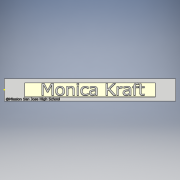
# Autodesk Inventor part: NameTag
Saved by Autodesk Inventor 2018 (Build 220112000, 112)
## iProperties
Created: 2019-03-18
Part Number: NameTag
Material: Generic
Document SubType Name: Modeling
Designer: This kid
Density: 1 g/cm^3
Appearance: Default
Author: This kid
Autodesk Inventor part; units mm, degrees
(part 1 of 2)
ref_plane "YZ Plane" through (0, 0, 0) normal (1, 0, 0) x (0, 1, 0)
ref_plane "XZ Plane" through (0, 0, 0) normal (0, 1, 0) x (-1, 0, 0)
ref_plane "XY Plane" through (0, 0, 0) normal (0, 0, 1) x (1, 0, 0)
sketch "Sketch1" plane through (0, 0, 0) normal (0, 0, 1) x (1, 0, 0)
  line L0 (0, 6.6514) -> (5.7603, -3.3257)
  line L1 (5.7603, -3.3257) -> (-5.7603, -3.3257)
  line L2 (-5.7603, -3.3257) -> (0, 6.6514)
  point P0 (0, 0)
  point P1 (0, 0)
  constraints: 6 end point, 1 coincident, 7 other
extrude "Extrusion1" add sketch "Sketch1" along normal blind 76.2
sketch "Sketch2" plane through (-5.7603, -3.3257, 0) normal (-0.8660254, 0.5, 0) x (0, 0, 1)
  line L0 (9.0292, 2.0917) -> (67.1704, 2.0917)
  line L1 (67.1704, 2.0917) -> (67.1704, 9.2481)
  line L2 (67.1704, 9.2481) -> (9.0292, 9.2481)
  line L3 (9.0292, 9.2481) -> (9.0292, 2.0917)
  line L4 (0, 5.7603) -> (9.0292, 5.6699) construction
  line L5 (67.1704, 5.7603) -> (76.2, 5.7603) construction
  constraints: 12 end point, 2 parallel, 1 equal length, 1 horizontal, 1 midpoint, 1 perpendicular, 1 point on line
extrude "Extrusion2" add sketch "Sketch2" along normal blind 0.2286
sketch "Sketch3" plane through (-5.9582, -3.2114, 0) normal (-0.8660254, 0.5, 0) x (0, 0, 1)
  point P0 (0, 5.7603)
sketch "Sketch4" plane through (-5.9582, -3.2114, 0) normal (-0.8660254, 0.5, 0) x (0, 0, 1)
  line L0 (9.8332, 9.129) -> (68.5929, 9.129) construction
  line L1 (68.5929, 9.129) -> (68.5929, 1.5104) construction
  line L2 (68.5929, 1.5104) -> (9.8332, 1.5104) construction
  line L3 (9.8332, 1.5104) -> (9.8332, 9.129) construction
  line L4 (21.8982, 2.7218) -> (21.0881, 2.7218)
  line L5 (21.0881, 2.7218) -> (21.0881, 7.9731)
  line L6 (21.0881, 7.9731) -> (19.4974, 4.4014)
  line L7 (19.4974, 4.4014) -> (19.0034, 4.4014)
  line L8 (19.0034, 4.4014) -> (17.4275, 7.9731)
  line L9 (17.4275, 7.9731) -> (17.4275, 2.7218)
  line L10 (17.4275, 2.7218) -> (16.6717, 2.7218)
  line L11 (16.6717, 2.7218) -> (16.6717, 8.8178)
  line L12 (16.6717, 8.8178) -> (17.7783, 8.8178)
  line L13 (17.7783, 8.8178) -> (19.2998, 5.424)
  line L14 (19.2998, 5.424) -> (20.7719, 8.8178)
  line L15 (20.7719, 8.8178) -> (21.8982, 8.8178)
  line L16 (21.8982, 8.8178) -> (21.8982, 2.7218)
  spline S0 degree 2 poles (26.8333, 5.009) (26.8333, 3.8531) (25.7218, 2.5934) (24.7931, 2.5934) knots 0 0 0 1 2 2 2
  spline S1 degree 2 poles (24.7931, 2.5934) (23.8397, 2.5934) (22.7479, 3.8926) (22.7479, 5.009) knots 0 0 0 1 2 2 2
  spline S2 degree 2 poles (22.7479, 5.009) (22.7479, 6.1551) (23.8743, 7.4247) (24.7931, 7.4247) knots 0 0 0 1 2 2 2
  spline S3 degree 2 poles (24.7931, 7.4247) (25.7218, 7.4247) (26.8333, 6.1601) (26.8333, 5.009) knots 0 0 0 1 2 2 2
  spline S4 degree 2 poles (26.038, 5.009) (26.038, 5.8983) (25.3908, 6.7628) (24.7931, 6.7628) knots 0 0 0 1 2 2 2
  spline S5 degree 2 poles (24.7931, 6.7628) (24.1954, 6.7628) (23.5433, 5.8983) (23.5433, 5.009) knots 0 0 0 1 2 2 2
  spline S6 degree 2 poles (23.5433, 5.009) (23.5433, 4.1445) (24.1954, 3.2553) (24.7931, 3.2553) knots 0 0 0 1 2 2 2
  spline S7 degree 2 poles (24.7931, 3.2553) (25.3859, 3.2553) (26.038, 4.1297) (26.038, 5.009) knots 0 0 0 1 2 2 2
  line L17 (31.2151, 2.7218) -> (30.4445, 2.7218)
  line L18 (30.4445, 2.7218) -> (30.4445, 5.3301)
  spline S8 degree 2 poles (30.4445, 5.3301) (30.4445, 5.6463) (30.3852, 6.1897) (30.2963, 6.3527) knots 0 0 0 1 2 2 2
  spline S9 degree 2 poles (30.2963, 6.3527) (30.2024, 6.5256) (29.8665, 6.6936) (29.58, 6.6936) knots 0 0 0 1 2 2 2
  spline S10 degree 2 poles (29.58, 6.6936) (29.2935, 6.6936) (28.6858, 6.3873) (28.3944, 6.1403) knots 0 0 0 1 2 2 2
  line L19 (28.3944, 6.1403) -> (28.3944, 2.7218)
  line L20 (28.3944, 2.7218) -> (27.6237, 2.7218)
  line L21 (27.6237, 2.7218) -> (27.6237, 7.2963)
  line L22 (27.6237, 7.2963) -> (28.3944, 7.2963)
  line L23 (28.3944, 7.2963) -> (28.3944, 6.7875)
  spline S11 degree 2 poles (28.3944, 6.7875) (28.7402, 7.0987) (29.4071, 7.4247) (29.7825, 7.4247) knots 0 0 0 1 2 2 2
  spline S12 degree 2 poles (29.7825, 7.4247) (30.4544, 7.4247) (31.2151, 6.5355) (31.2151, 5.6908) knots 0 0 0 1 2 2 2
  line L24 (31.2151, 5.6908) -> (31.2151, 2.7218)
  line L25 (33.0825, 2.7218) -> (32.3118, 2.7218)
  line L26 (32.3118, 2.7218) -> (32.3118, 7.2963)
  line L27 (32.3118, 7.2963) -> (33.0825, 7.2963)
  line L28 (33.0825, 7.2963) -> (33.0825, 2.7218)
  line L29 (33.1368, 8.057) -> (32.2624, 8.057)
  line L30 (32.2624, 8.057) -> (32.2624, 8.8573)
  line L31 (32.2624, 8.8573) -> (33.1368, 8.8573)
  line L32 (33.1368, 8.8573) -> (33.1368, 8.057)
  spline S13 degree 2 poles (36.0317, 2.6181) (35.5574, 2.6181) (34.772, 2.9095) (34.4904, 3.2059) knots 0 0 0 1 2 2 2
  spline S14 degree 2 poles (34.4904, 3.2059) (34.2088, 3.4974) (33.8976, 4.3965) (33.8976, 4.9992) knots 0 0 0 1 2 2 2
  spline S15 degree 2 poles (33.8976, 4.9992) (33.8976, 5.6019) (34.2187, 6.4812) (34.4904, 6.7776) knots 0 0 0 1 2 2 2
  spline S16 degree 2 poles (34.4904, 6.7776) (34.7621, 7.0789) (35.5673, 7.4) (36.0317, 7.4) knots 0 0 0 1 2 2 2
  spline S17 degree 2 poles (36.0317, 7.4) (36.4071, 7.4) (37.1086, 7.1876) (37.3803, 7.0493) knots 0 0 0 1 2 2 2
  line L33 (37.3803, 7.0493) -> (37.3803, 6.1848)
  line L34 (37.3803, 6.1848) -> (37.3358, 6.1848)
  spline S18 degree 2 poles (37.3358, 6.1848) (37.2519, 6.2539) (36.995, 6.4318) (36.8122, 6.5256) knots 0 0 0 1 2 2 2
  spline S19 degree 2 poles (36.8122, 6.5256) (36.6492, 6.6047) (36.2145, 6.7282) (36.0169, 6.7282) knots 0 0 0 1 2 2 2
  spline S20 degree 2 poles (36.0169, 6.7282) (35.4191, 6.7282) (34.6929, 5.8242) (34.6929, 4.9992) knots 0 0 0 1 2 2 2
  spline S21 degree 2 poles (34.6929, 4.9992) (34.6929, 4.1939) (35.3944, 3.2899) (36.0169, 3.2899) knots 0 0 0 1 2 2 2
  spline S22 degree 2 poles (36.0169, 3.2899) (36.3923, 3.2899) (37.074, 3.6011) (37.3358, 3.8432) knots 0 0 0 1 2 2 2
  line L35 (37.3358, 3.8432) -> (37.3803, 3.8432)
  line L36 (37.3803, 3.8432) -> (37.3803, 2.9787)
  spline S23 degree 2 poles (37.3803, 2.9787) (37.2667, 2.9244) (36.9209, 2.7712) (36.7826, 2.7366) knots 0 0 0 1 2 2 2
  spline S24 degree 2 poles (36.7826, 2.7366) (36.585, 2.6774) (36.2737, 2.6181) (36.0317, 2.6181) knots 0 0 0 1 2 2 2
  spline S25 degree 2 poles (40.6308, 3.2059) (40.537, 3.1368) (40.2208, 2.8898) (40.0726, 2.8157) knots 0 0 0 1 2 2 2
  spline S26 degree 2 poles (40.0726, 2.8157) (39.8701, 2.707) (39.4897, 2.5934) (39.1439, 2.5934) knots 0 0 0 1 2 2 2
  spline S27 degree 2 poles (39.1439, 2.5934) (38.8623, 2.5934) (38.3535, 2.8058) (38.1608, 2.9985) knots 0 0 0 1 2 2 2
  spline S28 degree 2 poles (38.1608, 2.9985) (37.978, 3.1862) (37.7557, 3.7395) (37.7557, 4.0457) knots 0 0 0 1 2 2 2
  spline S29 degree 2 poles (37.7557, 4.0457) (37.7557, 4.52) (38.1559, 5.1918) (38.5906, 5.3845) knots 0 0 0 1 2 2 2
  spline S30 degree 2 poles (38.5906, 5.3845) (38.9759, 5.5623) (40.0232, 5.6957) (40.6308, 5.7303) knots 0 0 0 1 2 2 2
  line L37 (40.6308, 5.7303) -> (40.6308, 5.8785)
  spline S31 degree 2 poles (40.6308, 5.8785) (40.6308, 6.1453) (40.4678, 6.4762) (40.3196, 6.5701) knots 0 0 0 1 2 2 2
  spline S32 degree 2 poles (40.3196, 6.5701) (40.1714, 6.664) (39.7466, 6.7232) (39.5193, 6.7232) knots 0 0 0 1 2 2 2
  spline S33 degree 2 poles (39.5193, 6.7232) (39.2526, 6.7232) (38.5313, 6.5652) (38.1707, 6.412) knots 0 0 0 1 2 2 2
  line L38 (38.1707, 6.412) -> (38.1263, 6.412)
  line L39 (38.1263, 6.412) -> (38.1263, 7.1975)
  spline S34 degree 2 poles (38.1263, 7.1975) (38.3387, 7.2568) (39.134, 7.405) (39.5243, 7.405) knots 0 0 0 1 2 2 2
  spline S35 degree 2 poles (39.5243, 7.405) (39.9985, 7.405) (40.6457, 7.2568) (40.9025, 7.0641) knots 0 0 0 1 2 2 2
  spline S36 degree 2 poles (40.9025, 7.0641) (41.1545, 6.8764) (41.4015, 6.2786) (41.4015, 5.8489) knots 0 0 0 1 2 2 2
  line L40 (41.4015, 5.8489) -> (41.4015, 2.7218)
  line L41 (41.4015, 2.7218) -> (40.6308, 2.7218)
  line L42 (40.6308, 2.7218) -> (40.6308, 3.2059)
  line L43 (40.6308, 3.8481) -> (40.6308, 5.1177)
  spline S37 degree 2 poles (40.6308, 5.1177) (40.3542, 5.093) (39.5193, 5.009) (39.2575, 4.93) knots 0 0 0 1 2 2 2
  spline S38 degree 2 poles (39.2575, 4.93) (38.9512, 4.8361) (38.5511, 4.4459) (38.5511, 4.1001) knots 0 0 0 1 2 2 2
  spline S39 degree 2 poles (38.5511, 4.1001) (38.5511, 3.7049) (38.9957, 3.3047) (39.4205, 3.3047) knots 0 0 0 1 2 2 2
  spline S40 degree 2 poles (39.4205, 3.3047) (39.7812, 3.3047) (40.374, 3.616) (40.6308, 3.8481) knots 0 0 0 1 2 2 2
  line L44 (49.6069, 2.7218) -> (48.5547, 2.7218)
  line L45 (48.5547, 2.7218) -> (46.3267, 5.5574)
  line L46 (46.3267, 5.5574) -> (45.971, 5.1572)
  line L47 (45.971, 5.1572) -> (45.971, 2.7218)
  line L48 (45.971, 2.7218) -> (45.1609, 2.7218)
  line L49 (45.1609, 2.7218) -> (45.1609, 8.8178)
  line L50 (45.1609, 8.8178) -> (45.971, 8.8178)
  line L51 (45.971, 8.8178) -> (45.971, 6.0168)
  line L52 (45.971, 6.0168) -> (48.4707, 8.8178)
  line L53 (48.4707, 8.8178) -> (49.4587, 8.8178)
  line L54 (49.4587, 8.8178) -> (46.9343, 6.0959)
  line L55 (46.9343, 6.0959) -> (49.6069, 2.7218)
  line L56 (52.4573, 6.4713) -> (52.4178, 6.4713)
  spline S41 degree 2 poles (52.4178, 6.4713) (52.3288, 6.496) (52.1362, 6.5059) (52.0028, 6.5059) knots 0 0 0 1 2 2 2
  spline S42 degree 2 poles (52.0028, 6.5059) (51.6916, 6.5059) (51.079, 6.2342) (50.8024, 5.9674) knots 0 0 0 1 2 2 2
  line L57 (50.8024, 5.9674) -> (50.8024, 2.7218)
  line L58 (50.8024, 2.7218) -> (50.0317, 2.7218)
  line L59 (50.0317, 2.7218) -> (50.0317, 7.2963)
  line L60 (50.0317, 7.2963) -> (50.8024, 7.2963)
  line L61 (50.8024, 7.2963) -> (50.8024, 6.6146)
  spline S43 degree 2 poles (50.8024, 6.6146) (51.2223, 6.99) (51.8497, 7.2963) (52.1461, 7.2963) knots 0 0 0 1 2 2 2
  spline S44 degree 2 poles (52.1461, 7.2963) (52.2646, 7.2963) (52.3832, 7.2864) (52.4573, 7.2716) knots 0 0 0 1 2 2 2
  line L62 (52.4573, 7.2716) -> (52.4573, 6.4713)
  spline S45 degree 2 poles (55.6041, 3.2059) (55.5102, 3.1368) (55.1941, 2.8898) (55.0459, 2.8157) knots 0 0 0 1 2 2 2
  spline S46 degree 2 poles (55.0459, 2.8157) (54.8433, 2.707) (54.4629, 2.5934) (54.1171, 2.5934) knots 0 0 0 1 2 2 2
  spline S47 degree 2 poles (54.1171, 2.5934) (53.8356, 2.5934) (53.3267, 2.8058) (53.1341, 2.9985) knots 0 0 0 1 2 2 2
  spline S48 degree 2 poles (53.1341, 2.9985) (52.9513, 3.1862) (52.729, 3.7395) (52.729, 4.0457) knots 0 0 0 1 2 2 2
  spline S49 degree 2 poles (52.729, 4.0457) (52.729, 4.52) (53.1291, 5.1918) (53.5639, 5.3845) knots 0 0 0 1 2 2 2
  spline S50 degree 2 poles (53.5639, 5.3845) (53.9492, 5.5623) (54.9965, 5.6957) (55.6041, 5.7303) knots 0 0 0 1 2 2 2
  line L63 (55.6041, 5.7303) -> (55.6041, 5.8785)
  spline S51 degree 2 poles (55.6041, 5.8785) (55.6041, 6.1453) (55.4411, 6.4762) (55.2929, 6.5701) knots 0 0 0 1 2 2 2
  spline S52 degree 2 poles (55.2929, 6.5701) (55.1447, 6.664) (54.7198, 6.7232) (54.4926, 6.7232) knots 0 0 0 1 2 2 2
  spline S53 degree 2 poles (54.4926, 6.7232) (54.2258, 6.7232) (53.5046, 6.5652) (53.1439, 6.412) knots 0 0 0 1 2 2 2
  line L64 (53.1439, 6.412) -> (53.0995, 6.412)
  line L65 (53.0995, 6.412) -> (53.0995, 7.1975)
  spline S54 degree 2 poles (53.0995, 7.1975) (53.3119, 7.2568) (54.1073, 7.405) (54.4975, 7.405) knots 0 0 0 1 2 2 2
  spline S55 degree 2 poles (54.4975, 7.405) (54.9718, 7.405) (55.6189, 7.2568) (55.8758, 7.0641) knots 0 0 0 1 2 2 2
  spline S56 degree 2 poles (55.8758, 7.0641) (56.1277, 6.8764) (56.3747, 6.2786) (56.3747, 5.8489) knots 0 0 0 1 2 2 2
  line L66 (56.3747, 5.8489) -> (56.3747, 2.7218)
  line L67 (56.3747, 2.7218) -> (55.6041, 2.7218)
  line L68 (55.6041, 2.7218) -> (55.6041, 3.2059)
  line L69 (55.6041, 3.8481) -> (55.6041, 5.1177)
  spline S57 degree 2 poles (55.6041, 5.1177) (55.3274, 5.093) (54.4926, 5.009) (54.2308, 4.93) knots 0 0 0 1 2 2 2
  spline S58 degree 2 poles (54.2308, 4.93) (53.9245, 4.8361) (53.5243, 4.4459) (53.5243, 4.1001) knots 0 0 0 1 2 2 2
  spline S59 degree 2 poles (53.5243, 4.1001) (53.5243, 3.7049) (53.9689, 3.3047) (54.3938, 3.3047) knots 0 0 0 1 2 2 2
  spline S60 degree 2 poles (54.3938, 3.3047) (54.7544, 3.3047) (55.3472, 3.616) (55.6041, 3.8481) knots 0 0 0 1 2 2 2
  line L70 (59.8624, 8.3485) -> (59.8229, 8.3485)
  spline S61 degree 2 poles (59.8229, 8.3485) (59.7191, 8.388) (59.3338, 8.4572) (59.1807, 8.4572) knots 0 0 0 1 2 2 2
  spline S62 degree 2 poles (59.1807, 8.4572) (58.6965, 8.4572) (58.2816, 8.0225) (58.2816, 7.4494) knots 0 0 0 1 2 2 2
  line L71 (58.2816, 7.4494) -> (58.2816, 7.2963)
  line L72 (58.2816, 7.2963) -> (59.5561, 7.2963)
  line L73 (59.5561, 7.2963) -> (59.5561, 6.659)
  line L74 (59.5561, 6.659) -> (58.3063, 6.659)
  line L75 (58.3063, 6.659) -> (58.3063, 2.7218)
  line L76 (58.3063, 2.7218) -> (57.5356, 2.7218)
  line L77 (57.5356, 2.7218) -> (57.5356, 6.659)
  line L78 (57.5356, 6.659) -> (57.0169, 6.659)
  line L79 (57.0169, 6.659) -> (57.0169, 7.2963)
  line L80 (57.0169, 7.2963) -> (57.5356, 7.2963)
  line L81 (57.5356, 7.2963) -> (57.5356, 7.4494)
  spline S63 degree 2 poles (57.5356, 7.4494) (57.5356, 8.2695) (58.331, 9.129) (59.072, 9.129) knots 0 0 0 1 2 2 2
  spline S64 degree 2 poles (59.072, 9.129) (59.2844, 9.129) (59.6944, 9.0846) (59.8624, 9.0549) knots 0 0 0 1 2 2 2
  line L82 (59.8624, 9.0549) -> (59.8624, 8.3485)
  spline S65 degree 2 poles (61.5074, 2.6329) (60.88, 2.6329) (60.1736, 3.3492) (60.1736, 4.1248) knots 0 0 0 1 2 2 2
  line L83 (60.1736, 4.1248) -> (60.1736, 6.659)
  line L84 (60.1736, 6.659) -> (59.6549, 6.659)
  line L85 (59.6549, 6.659) -> (59.6549, 7.2963)
  line L86 (59.6549, 7.2963) -> (60.1736, 7.2963)
  line L87 (60.1736, 7.2963) -> (60.1736, 8.6103)
  line L88 (60.1736, 8.6103) -> (60.9443, 8.6103)
  line L89 (60.9443, 8.6103) -> (60.9443, 7.2963)
  line L90 (60.9443, 7.2963) -> (62.362, 7.2963)
  line L91 (62.362, 7.2963) -> (62.362, 6.659)
  line L92 (62.362, 6.659) -> (60.9443, 6.659)
  line L93 (60.9443, 6.659) -> (60.9443, 4.4805)
  spline S66 degree 2 poles (60.9443, 4.4805) (60.9443, 4.1347) (60.969, 3.7543) (61.0529, 3.5913) knots 0 0 0 1 2 2 2
  spline S67 degree 2 poles (61.0529, 3.5913) (61.1221, 3.448) (61.4333, 3.3047) (61.7001, 3.3047) knots 0 0 0 1 2 2 2
  spline S68 degree 2 poles (61.7001, 3.3047) (61.8878, 3.3047) (62.2385, 3.4184) (62.3176, 3.4529) knots 0 0 0 1 2 2 2
  line L94 (62.3176, 3.4529) -> (62.362, 3.4529)
  line L95 (62.362, 3.4529) -> (62.362, 2.7613)
  spline S69 degree 2 poles (62.362, 2.7613) (62.1447, 2.7021) (61.7001, 2.6329) (61.5074, 2.6329) knots 0 0 0 1 2 2 2
  point P0 (0, 5.7603)
  constraints: 2 other
extrude "Extrusion3" add sketch "Sketch4" along normal blind 0.254
sketch "Sketch5" plane through (0, 6.6514, 76.2) normal (0.8660254, 0.5, 0) x (0, 0, -1)
  line L0 (67.0697, -2.2328) -> (67.0697, -9.3892)
  line L1 (9.3366, -9.3892) -> (67.0697, -9.3892)
  line L2 (67.0697, -2.2328) -> (9.3366, -2.2328)
  line L3 (9.3366, -2.2328) -> (9.3366, -9.3892)
  line L4 (67.0697, -5.811) -> (76.4063, -5.811) construction
  line L5 (0, -5.7603) -> (9.3366, -5.7603) construction
  constraints: 12 end point, 1 horizontal, 1 midpoint, 1 parallel, 1 perpendicular, 1 point on line, 1 vertical
extrude "Extrusion4" add sketch "Sketch5" along normal blind 0.2286
sketch "Sketch6" plane through (0.198, 6.7657, 76.2) normal (0.8660254, 0.5, 0) x (0, 0, -1)
  line L0 (9.5837, -2.534) -> (68.3434, -2.534) construction
  line L1 (68.3434, -2.534) -> (68.3434, -8.4681) construction
  line L2 (68.3434, -8.4681) -> (9.5837, -8.4681) construction
  line L3 (9.5837, -8.4681) -> (9.5837, -2.534) construction
  line L4 (21.6488, -8.9412) -> (20.8386, -8.9412)
  line L5 (20.8386, -8.9412) -> (20.8386, -3.69)
  line L6 (20.8386, -3.69) -> (19.2479, -7.2616)
  line L7 (19.2479, -7.2616) -> (18.7539, -7.2616)
  line L8 (18.7539, -7.2616) -> (17.1781, -3.69)
  line L9 (17.1781, -3.69) -> (17.1781, -8.9412)
  line L10 (17.1781, -8.9412) -> (16.4222, -8.9412)
  line L11 (16.4222, -8.9412) -> (16.4222, -2.8452)
  line L12 (16.4222, -2.8452) -> (17.5288, -2.8452)
  line L13 (17.5288, -2.8452) -> (19.0503, -6.239)
  line L14 (19.0503, -6.239) -> (20.5225, -2.8452)
  line L15 (20.5225, -2.8452) -> (21.6488, -2.8452)
  line L16 (21.6488, -2.8452) -> (21.6488, -8.9412)
  spline S0 degree 2 poles (26.5839, -6.654) (26.5839, -7.81) (25.4724, -9.0697) (24.5436, -9.0697) knots 0 0 0 1 2 2 2
  spline S1 degree 2 poles (24.5436, -9.0697) (23.5902, -9.0697) (22.4985, -7.7704) (22.4985, -6.654) knots 0 0 0 1 2 2 2
  spline S2 degree 2 poles (22.4985, -6.654) (22.4985, -5.5079) (23.6248, -4.2383) (24.5436, -4.2383) knots 0 0 0 1 2 2 2
  spline S3 degree 2 poles (24.5436, -4.2383) (25.4724, -4.2383) (26.5839, -5.503) (26.5839, -6.654) knots 0 0 0 1 2 2 2
  spline S4 degree 2 poles (25.7885, -6.654) (25.7885, -5.7648) (25.1414, -4.9003) (24.5436, -4.9003) knots 0 0 0 1 2 2 2
  spline S5 degree 2 poles (24.5436, -4.9003) (23.9459, -4.9003) (23.2938, -5.7648) (23.2938, -6.654) knots 0 0 0 1 2 2 2
  spline S6 degree 2 poles (23.2938, -6.654) (23.2938, -7.5185) (23.9459, -8.4077) (24.5436, -8.4077) knots 0 0 0 1 2 2 2
  spline S7 degree 2 poles (24.5436, -8.4077) (25.1364, -8.4077) (25.7885, -7.5333) (25.7885, -6.654) knots 0 0 0 1 2 2 2
  line L17 (30.9657, -8.9412) -> (30.195, -8.9412)
  line L18 (30.195, -8.9412) -> (30.195, -6.3329)
  spline S8 degree 2 poles (30.195, -6.3329) (30.195, -6.0167) (30.1358, -5.4733) (30.0468, -5.3103) knots 0 0 0 1 2 2 2
  spline S9 degree 2 poles (30.0468, -5.3103) (29.953, -5.1374) (29.6171, -4.9694) (29.3305, -4.9694) knots 0 0 0 1 2 2 2
  spline S10 degree 2 poles (29.3305, -4.9694) (29.044, -4.9694) (28.4364, -5.2757) (28.1449, -5.5227) knots 0 0 0 1 2 2 2
  line L19 (28.1449, -5.5227) -> (28.1449, -8.9412)
  line L20 (28.1449, -8.9412) -> (27.3743, -8.9412)
  line L21 (27.3743, -8.9412) -> (27.3743, -4.3668)
  line L22 (27.3743, -4.3668) -> (28.1449, -4.3668)
  line L23 (28.1449, -4.3668) -> (28.1449, -4.8756)
  spline S11 degree 2 poles (28.1449, -4.8756) (28.4907, -4.5644) (29.1576, -4.2383) (29.5331, -4.2383) knots 0 0 0 1 2 2 2
  spline S12 degree 2 poles (29.5331, -4.2383) (30.2049, -4.2383) (30.9657, -5.1275) (30.9657, -5.9723) knots 0 0 0 1 2 2 2
  line L24 (30.9657, -5.9723) -> (30.9657, -8.9412)
  line L25 (32.833, -8.9412) -> (32.0624, -8.9412)
  line L26 (32.0624, -8.9412) -> (32.0624, -4.3668)
  line L27 (32.0624, -4.3668) -> (32.833, -4.3668)
  line L28 (32.833, -4.3668) -> (32.833, -8.9412)
  line L29 (32.8874, -3.606) -> (32.013, -3.606)
  line L30 (32.013, -3.606) -> (32.013, -2.8057)
  line L31 (32.013, -2.8057) -> (32.8874, -2.8057)
  line L32 (32.8874, -2.8057) -> (32.8874, -3.606)
  spline S13 degree 2 poles (35.7822, -9.045) (35.308, -9.045) (34.5225, -8.7535) (34.2409, -8.4571) knots 0 0 0 1 2 2 2
  spline S14 degree 2 poles (34.2409, -8.4571) (33.9593, -8.1656) (33.6481, -7.2666) (33.6481, -6.6639) knots 0 0 0 1 2 2 2
  spline S15 degree 2 poles (33.6481, -6.6639) (33.6481, -6.0612) (33.9692, -5.1819) (34.2409, -4.8855) knots 0 0 0 1 2 2 2
  spline S16 degree 2 poles (34.2409, -4.8855) (34.5126, -4.5841) (35.3179, -4.263) (35.7822, -4.263) knots 0 0 0 1 2 2 2
  spline S17 degree 2 poles (35.7822, -4.263) (36.1577, -4.263) (36.8591, -4.4754) (37.1308, -4.6138) knots 0 0 0 1 2 2 2
  line L33 (37.1308, -4.6138) -> (37.1308, -5.4783)
  line L34 (37.1308, -5.4783) -> (37.0864, -5.4783)
  spline S18 degree 2 poles (37.0864, -5.4783) (37.0024, -5.4091) (36.7455, -5.2313) (36.5627, -5.1374) knots 0 0 0 1 2 2 2
  spline S19 degree 2 poles (36.5627, -5.1374) (36.3997, -5.0584) (35.965, -4.9349) (35.7674, -4.9349) knots 0 0 0 1 2 2 2
  spline S20 degree 2 poles (35.7674, -4.9349) (35.1697, -4.9349) (34.4435, -5.8389) (34.4435, -6.6639) knots 0 0 0 1 2 2 2
  spline S21 degree 2 poles (34.4435, -6.6639) (34.4435, -7.4691) (35.145, -8.3731) (35.7674, -8.3731) knots 0 0 0 1 2 2 2
  spline S22 degree 2 poles (35.7674, -8.3731) (36.1428, -8.3731) (36.8246, -8.0619) (37.0864, -7.8198) knots 0 0 0 1 2 2 2
  line L35 (37.0864, -7.8198) -> (37.1308, -7.8198)
  line L36 (37.1308, -7.8198) -> (37.1308, -8.6843)
  spline S23 degree 2 poles (37.1308, -8.6843) (37.0172, -8.7387) (36.6714, -8.8918) (36.5331, -8.9264) knots 0 0 0 1 2 2 2
  spline S24 degree 2 poles (36.5331, -8.9264) (36.3355, -8.9857) (36.0243, -9.045) (35.7822, -9.045) knots 0 0 0 1 2 2 2
  spline S25 degree 2 poles (40.3814, -8.4571) (40.2875, -8.5263) (39.9714, -8.7733) (39.8232, -8.8474) knots 0 0 0 1 2 2 2
  spline S26 degree 2 poles (39.8232, -8.8474) (39.6206, -8.9561) (39.2402, -9.0697) (38.8944, -9.0697) knots 0 0 0 1 2 2 2
  spline S27 degree 2 poles (38.8944, -9.0697) (38.6129, -9.0697) (38.104, -8.8573) (37.9114, -8.6646) knots 0 0 0 1 2 2 2
  spline S28 degree 2 poles (37.9114, -8.6646) (37.7286, -8.4769) (37.5063, -7.9236) (37.5063, -7.6173) knots 0 0 0 1 2 2 2
  spline S29 degree 2 poles (37.5063, -7.6173) (37.5063, -7.1431) (37.9064, -6.4712) (38.3412, -6.2786) knots 0 0 0 1 2 2 2
  spline S30 degree 2 poles (38.3412, -6.2786) (38.7265, -6.1007) (39.7738, -5.9673) (40.3814, -5.9328) knots 0 0 0 1 2 2 2
  line L37 (40.3814, -5.9328) -> (40.3814, -5.7846)
  spline S31 degree 2 poles (40.3814, -5.7846) (40.3814, -5.5178) (40.2184, -5.1868) (40.0702, -5.0929) knots 0 0 0 1 2 2 2
  spline S32 degree 2 poles (40.0702, -5.0929) (39.922, -4.9991) (39.4971, -4.9398) (39.2699, -4.9398) knots 0 0 0 1 2 2 2
  spline S33 degree 2 poles (39.2699, -4.9398) (39.0031, -4.9398) (38.2819, -5.0979) (37.9212, -5.251) knots 0 0 0 1 2 2 2
  line L38 (37.9212, -5.251) -> (37.8768, -5.251)
  line L39 (37.8768, -5.251) -> (37.8768, -4.4656)
  spline S34 degree 2 poles (37.8768, -4.4656) (38.0892, -4.4063) (38.8846, -4.2581) (39.2748, -4.2581) knots 0 0 0 1 2 2 2
  spline S35 degree 2 poles (39.2748, -4.2581) (39.7491, -4.2581) (40.3962, -4.4063) (40.6531, -4.5989) knots 0 0 0 1 2 2 2
  spline S36 degree 2 poles (40.6531, -4.5989) (40.905, -4.7867) (41.152, -5.3844) (41.152, -5.8142) knots 0 0 0 1 2 2 2
  line L40 (41.152, -5.8142) -> (41.152, -8.9412)
  line L41 (41.152, -8.9412) -> (40.3814, -8.9412)
  line L42 (40.3814, -8.9412) -> (40.3814, -8.4571)
  line L43 (40.3814, -7.8149) -> (40.3814, -6.5453)
  spline S37 degree 2 poles (40.3814, -6.5453) (40.1047, -6.57) (39.2699, -6.654) (39.0081, -6.733) knots 0 0 0 1 2 2 2
  spline S38 degree 2 poles (39.0081, -6.733) (38.7018, -6.8269) (38.3016, -7.2172) (38.3016, -7.563) knots 0 0 0 1 2 2 2
  spline S39 degree 2 poles (38.3016, -7.563) (38.3016, -7.9582) (38.7462, -8.3583) (39.1711, -8.3583) knots 0 0 0 1 2 2 2
  spline S40 degree 2 poles (39.1711, -8.3583) (39.5317, -8.3583) (40.1245, -8.0471) (40.3814, -7.8149) knots 0 0 0 1 2 2 2
  line L44 (49.3574, -8.9412) -> (48.3052, -8.9412)
  line L45 (48.3052, -8.9412) -> (46.0772, -6.1057)
  line L46 (46.0772, -6.1057) -> (45.7216, -6.5058)
  line L47 (45.7216, -6.5058) -> (45.7216, -8.9412)
  line L48 (45.7216, -8.9412) -> (44.9114, -8.9412)
  line L49 (44.9114, -8.9412) -> (44.9114, -2.8452)
  line L50 (44.9114, -2.8452) -> (45.7216, -2.8452)
  line L51 (45.7216, -2.8452) -> (45.7216, -5.6462)
  line L52 (45.7216, -5.6462) -> (48.2212, -2.8452)
  line L53 (48.2212, -2.8452) -> (49.2092, -2.8452)
  line L54 (49.2092, -2.8452) -> (46.6849, -5.5672)
  line L55 (46.6849, -5.5672) -> (49.3574, -8.9412)
  line L56 (52.2078, -5.1917) -> (52.1683, -5.1917)
  spline S41 degree 2 poles (52.1683, -5.1917) (52.0794, -5.167) (51.8867, -5.1572) (51.7533, -5.1572) knots 0 0 0 1 2 2 2
  spline S42 degree 2 poles (51.7533, -5.1572) (51.4421, -5.1572) (50.8296, -5.4289) (50.5529, -5.6956) knots 0 0 0 1 2 2 2
  line L57 (50.5529, -5.6956) -> (50.5529, -8.9412)
  line L58 (50.5529, -8.9412) -> (49.7823, -8.9412)
  line L59 (49.7823, -8.9412) -> (49.7823, -4.3668)
  line L60 (49.7823, -4.3668) -> (50.5529, -4.3668)
  line L61 (50.5529, -4.3668) -> (50.5529, -5.0485)
  spline S43 degree 2 poles (50.5529, -5.0485) (50.9728, -4.673) (51.6002, -4.3668) (51.8966, -4.3668) knots 0 0 0 1 2 2 2
  spline S44 degree 2 poles (51.8966, -4.3668) (52.0152, -4.3668) (52.1337, -4.3766) (52.2078, -4.3915) knots 0 0 0 1 2 2 2
  line L62 (52.2078, -4.3915) -> (52.2078, -5.1917)
  spline S45 degree 2 poles (55.3546, -8.4571) (55.2608, -8.5263) (54.9446, -8.7733) (54.7964, -8.8474) knots 0 0 0 1 2 2 2
  spline S46 degree 2 poles (54.7964, -8.8474) (54.5939, -8.9561) (54.2135, -9.0697) (53.8677, -9.0697) knots 0 0 0 1 2 2 2
  spline S47 degree 2 poles (53.8677, -9.0697) (53.5861, -9.0697) (53.0773, -8.8573) (52.8846, -8.6646) knots 0 0 0 1 2 2 2
  spline S48 degree 2 poles (52.8846, -8.6646) (52.7018, -8.4769) (52.4795, -7.9236) (52.4795, -7.6173) knots 0 0 0 1 2 2 2
  spline S49 degree 2 poles (52.4795, -7.6173) (52.4795, -7.1431) (52.8797, -6.4712) (53.3144, -6.2786) knots 0 0 0 1 2 2 2
  spline S50 degree 2 poles (53.3144, -6.2786) (53.6997, -6.1007) (54.747, -5.9673) (55.3546, -5.9328) knots 0 0 0 1 2 2 2
  line L63 (55.3546, -5.9328) -> (55.3546, -5.7846)
  spline S51 degree 2 poles (55.3546, -5.7846) (55.3546, -5.5178) (55.1916, -5.1868) (55.0434, -5.0929) knots 0 0 0 1 2 2 2
  spline S52 degree 2 poles (55.0434, -5.0929) (54.8952, -4.9991) (54.4704, -4.9398) (54.2431, -4.9398) knots 0 0 0 1 2 2 2
  spline S53 degree 2 poles (54.2431, -4.9398) (53.9764, -4.9398) (53.2551, -5.0979) (52.8945, -5.251) knots 0 0 0 1 2 2 2
  line L64 (52.8945, -5.251) -> (52.85, -5.251)
  line L65 (52.85, -5.251) -> (52.85, -4.4656)
  spline S54 degree 2 poles (52.85, -4.4656) (53.0624, -4.4063) (53.8578, -4.2581) (54.2481, -4.2581) knots 0 0 0 1 2 2 2
  spline S55 degree 2 poles (54.2481, -4.2581) (54.7223, -4.2581) (55.3694, -4.4063) (55.6263, -4.5989) knots 0 0 0 1 2 2 2
  spline S56 degree 2 poles (55.6263, -4.5989) (55.8783, -4.7867) (56.1253, -5.3844) (56.1253, -5.8142) knots 0 0 0 1 2 2 2
  line L66 (56.1253, -5.8142) -> (56.1253, -8.9412)
  line L67 (56.1253, -8.9412) -> (55.3546, -8.9412)
  line L68 (55.3546, -8.9412) -> (55.3546, -8.4571)
  line L69 (55.3546, -7.8149) -> (55.3546, -6.5453)
  spline S57 degree 2 poles (55.3546, -6.5453) (55.078, -6.57) (54.2431, -6.654) (53.9813, -6.733) knots 0 0 0 1 2 2 2
  spline S58 degree 2 poles (53.9813, -6.733) (53.675, -6.8269) (53.2749, -7.2172) (53.2749, -7.563) knots 0 0 0 1 2 2 2
  spline S59 degree 2 poles (53.2749, -7.563) (53.2749, -7.9582) (53.7195, -8.3583) (54.1443, -8.3583) knots 0 0 0 1 2 2 2
  spline S60 degree 2 poles (54.1443, -8.3583) (54.5049, -8.3583) (55.0977, -8.0471) (55.3546, -7.8149) knots 0 0 0 1 2 2 2
  line L70 (59.6129, -3.3145) -> (59.5734, -3.3145)
  spline S61 degree 2 poles (59.5734, -3.3145) (59.4697, -3.275) (59.0843, -3.2059) (58.9312, -3.2059) knots 0 0 0 1 2 2 2
  spline S62 degree 2 poles (58.9312, -3.2059) (58.4471, -3.2059) (58.0321, -3.6406) (58.0321, -4.2136) knots 0 0 0 1 2 2 2
  line L71 (58.0321, -4.2136) -> (58.0321, -4.3668)
  line L72 (58.0321, -4.3668) -> (59.3066, -4.3668)
  line L73 (59.3066, -4.3668) -> (59.3066, -5.004)
  line L74 (59.3066, -5.004) -> (58.0568, -5.004)
  line L75 (58.0568, -5.004) -> (58.0568, -8.9412)
  line L76 (58.0568, -8.9412) -> (57.2862, -8.9412)
  line L77 (57.2862, -8.9412) -> (57.2862, -5.004)
  line L78 (57.2862, -5.004) -> (56.7675, -5.004)
  line L79 (56.7675, -5.004) -> (56.7675, -4.3668)
  line L80 (56.7675, -4.3668) -> (57.2862, -4.3668)
  line L81 (57.2862, -4.3668) -> (57.2862, -4.2136)
  spline S63 degree 2 poles (57.2862, -4.2136) (57.2862, -3.3936) (58.0815, -2.534) (58.8225, -2.534) knots 0 0 0 1 2 2 2
  spline S64 degree 2 poles (58.8225, -2.534) (59.0349, -2.534) (59.445, -2.5785) (59.6129, -2.6081) knots 0 0 0 1 2 2 2
  line L82 (59.6129, -2.6081) -> (59.6129, -3.3145)
  spline S65 degree 2 poles (61.258, -9.0302) (60.6306, -9.0302) (59.9242, -8.3138) (59.9242, -7.5383) knots 0 0 0 1 2 2 2
  line L83 (59.9242, -7.5383) -> (59.9242, -5.004)
  line L84 (59.9242, -5.004) -> (59.4055, -5.004)
  line L85 (59.4055, -5.004) -> (59.4055, -4.3668)
  line L86 (59.4055, -4.3668) -> (59.9242, -4.3668)
  line L87 (59.9242, -4.3668) -> (59.9242, -3.0527)
  line L88 (59.9242, -3.0527) -> (60.6948, -3.0527)
  line L89 (60.6948, -3.0527) -> (60.6948, -4.3668)
  line L90 (60.6948, -4.3668) -> (62.1126, -4.3668)
  line L91 (62.1126, -4.3668) -> (62.1126, -5.004)
  line L92 (62.1126, -5.004) -> (60.6948, -5.004)
  line L93 (60.6948, -5.004) -> (60.6948, -7.1826)
  spline S66 degree 2 poles (60.6948, -7.1826) (60.6948, -7.5284) (60.7195, -7.9088) (60.8035, -8.0718) knots 0 0 0 1 2 2 2
  spline S67 degree 2 poles (60.8035, -8.0718) (60.8726, -8.215) (61.1839, -8.3583) (61.4506, -8.3583) knots 0 0 0 1 2 2 2
  spline S68 degree 2 poles (61.4506, -8.3583) (61.6383, -8.3583) (61.9891, -8.2447) (62.0681, -8.2101) knots 0 0 0 1 2 2 2
  line L94 (62.0681, -8.2101) -> (62.1126, -8.2101)
  line L95 (62.1126, -8.2101) -> (62.1126, -8.9017)
  spline S69 degree 2 poles (62.1126, -8.9017) (61.8952, -8.961) (61.4506, -9.0302) (61.258, -9.0302) knots 0 0 0 1 2 2 2
  point P0 (76.2, -5.7603)
  point P1 (0, 5.7603)
  constraints: 2 other
extrude "Extrusion5" add sketch "Sketch6" along normal blind 0.2286
sketch "Sketch7" plane through (-5.7603, -3.3257, 0) normal (-0.8660254, 0.5, 0) x (0, 0, 1)
  line L0 (0.5735, 1.7459) -> (40.1435, 1.7459) construction
  line L1 (40.1435, 1.7459) -> (40.1435, 0.1688) construction
  line L2 (40.1435, 0.1688) -> (0.5735, 0.1688) construction
  line L3 (0.5735, 0.1688) -> (0.5735, 1.7459) construction
  spline S0 degree 2 poles (2.0565, 0.9853) (2.0565, 0.867) (1.9917, 0.6457) (1.931, 0.5541) knots 0 0 0 1 2 2 2
  line L4 (1.931, 0.5541) -> (1.5728, 0.5541)
  line L5 (1.5728, 0.5541) -> (1.5512, 0.6529)
  spline S1 degree 2 poles (1.5512, 0.6529) (1.4936, 0.6045) (1.3978, 0.5469) (1.3145, 0.5469) knots 0 0 0 1 2 2 2
  spline S2 degree 2 poles (1.3145, 0.5469) (1.1838, 0.5469) (1.016, 0.7579) (1.016, 0.9576) knots 0 0 0 1 2 2 2
  spline S3 degree 2 poles (1.016, 0.9576) (1.016, 1.1582) (1.2219, 1.3816) (1.3546, 1.3816) knots 0 0 0 1 2 2 2
  spline S4 degree 2 poles (1.3546, 1.3816) (1.4164, 1.3816) (1.5049, 1.3507) (1.5502, 1.325) knots 0 0 0 1 2 2 2
  line L6 (1.5502, 1.325) -> (1.5502, 1.3661)
  line L7 (1.5502, 1.3661) -> (1.685, 1.3661)
  line L8 (1.685, 1.3661) -> (1.685, 0.6488)
  line L9 (1.685, 0.6488) -> (1.8785, 0.6488)
  spline S5 degree 2 poles (1.8785, 0.6488) (1.9114, 0.7095) (1.9392, 0.902) (1.9392, 0.9802) knots 0 0 0 1 2 2 2
  spline S6 degree 2 poles (1.9392, 0.9802) (1.9392, 1.2591) (1.6551, 1.5987) (1.3886, 1.5987) knots 0 0 0 1 2 2 2
  spline S7 degree 2 poles (1.3886, 1.5987) (1.1364, 1.5987) (0.8081, 1.2313) (0.8081, 0.9689) knots 0 0 0 1 2 2 2
  spline S8 degree 2 poles (0.8081, 0.9689) (0.8081, 0.6879) (1.1272, 0.339) (1.3845, 0.339) knots 0 0 0 1 2 2 2
  spline S9 degree 2 poles (1.3845, 0.339) (1.4534, 0.339) (1.6068, 0.3575) (1.6747, 0.3781) knots 0 0 0 1 2 2 2
  line L10 (1.6747, 0.3781) -> (1.6747, 0.2577)
  spline S10 degree 2 poles (1.6747, 0.2577) (1.6027, 0.2402) (1.4555, 0.2268) (1.3834, 0.2268) knots 0 0 0 1 2 2 2
  spline S11 degree 2 poles (1.3834, 0.2268) (1.0819, 0.2268) (0.6857, 0.6416) (0.6857, 0.9709) knots 0 0 0 1 2 2 2
  spline S12 degree 2 poles (0.6857, 0.9709) (0.6857, 1.2838) (1.0942, 1.714) (1.3876, 1.714) knots 0 0 0 1 2 2 2
  spline S13 degree 2 poles (1.3876, 1.714) (1.7015, 1.714) (2.0565, 1.3095) (2.0565, 0.9853) knots 0 0 0 1 2 2 2
  line L11 (1.5481, 0.7672) -> (1.5481, 1.2087)
  spline S14 degree 2 poles (1.5481, 1.2087) (1.5008, 1.2334) (1.4205, 1.255) (1.3762, 1.255) knots 0 0 0 1 2 2 2
  spline S15 degree 2 poles (1.3762, 1.255) (1.2795, 1.255) (1.1622, 1.1109) (1.1622, 0.9596) knots 0 0 0 1 2 2 2
  spline S16 degree 2 poles (1.1622, 0.9596) (1.1622, 0.8238) (1.2507, 0.6786) (1.3484, 0.6786) knots 0 0 0 1 2 2 2
  spline S17 degree 2 poles (1.3484, 0.6786) (1.3999, 0.6786) (1.5018, 0.728) (1.5481, 0.7672) knots 0 0 0 1 2 2 2
  line L12 (3.379, 0.4193) -> (3.2102, 0.4193)
  line L13 (3.2102, 0.4193) -> (3.2102, 1.5133)
  line L14 (3.2102, 1.5133) -> (2.8788, 0.7692)
  line L15 (2.8788, 0.7692) -> (2.7759, 0.7692)
  line L16 (2.7759, 0.7692) -> (2.4476, 1.5133)
  line L17 (2.4476, 1.5133) -> (2.4476, 0.4193)
  line L18 (2.4476, 0.4193) -> (2.2901, 0.4193)
  line L19 (2.2901, 0.4193) -> (2.2901, 1.6893)
  line L20 (2.2901, 1.6893) -> (2.5207, 1.6893)
  line L21 (2.5207, 1.6893) -> (2.8377, 0.9823)
  line L22 (2.8377, 0.9823) -> (3.1444, 1.6893)
  line L23 (3.1444, 1.6893) -> (3.379, 1.6893)
  line L24 (3.379, 1.6893) -> (3.379, 0.4193)
  line L25 (3.7876, 0.4193) -> (3.627, 0.4193)
  line L26 (3.627, 0.4193) -> (3.627, 1.3723)
  line L27 (3.627, 1.3723) -> (3.7876, 1.3723)
  line L28 (3.7876, 1.3723) -> (3.7876, 0.4193)
  line L29 (3.7989, 1.5308) -> (3.6167, 1.5308)
  line L30 (3.6167, 1.5308) -> (3.6167, 1.6975)
  line L31 (3.6167, 1.6975) -> (3.7989, 1.6975)
  line L32 (3.7989, 1.6975) -> (3.7989, 1.5308)
  spline S18 degree 2 poles (4.2806, 0.3967) (4.1848, 0.3967) (4.0192, 0.4481) (3.9646, 0.4769) knots 0 0 0 1 2 2 2
  line L33 (3.9646, 0.4769) -> (3.9646, 0.657)
  line L34 (3.9646, 0.657) -> (3.9728, 0.657)
  spline S19 degree 2 poles (3.9728, 0.657) (3.9934, 0.6406) (4.049, 0.6015) (4.0953, 0.5798) knots 0 0 0 1 2 2 2
  spline S20 degree 2 poles (4.0953, 0.5798) (4.1354, 0.5603) (4.2342, 0.5315) (4.2867, 0.5315) knots 0 0 0 1 2 2 2
  spline S21 degree 2 poles (4.2867, 0.5315) (4.3248, 0.5315) (4.4123, 0.549) (4.4329, 0.5634) knots 0 0 0 1 2 2 2
  spline S22 degree 2 poles (4.4329, 0.5634) (4.4627, 0.5829) (4.4895, 0.6272) (4.4895, 0.6725) knots 0 0 0 1 2 2 2
  spline S23 degree 2 poles (4.4895, 0.6725) (4.4895, 0.7291) (4.4277, 0.7877) (4.3485, 0.8073) knots 0 0 0 1 2 2 2
  spline S24 degree 2 poles (4.3485, 0.8073) (4.3176, 0.8145) (4.2188, 0.8351) (4.1766, 0.8464) knots 0 0 0 1 2 2 2
  spline S25 degree 2 poles (4.1766, 0.8464) (4.0675, 0.8783) (3.9687, 1.01) (3.9687, 1.1037) knots 0 0 0 1 2 2 2
  spline S26 degree 2 poles (3.9687, 1.1037) (3.9687, 1.2334) (4.1632, 1.395) (4.3238, 1.395) knots 0 0 0 1 2 2 2
  spline S27 degree 2 poles (4.3238, 1.395) (4.403, 1.395) (4.5636, 1.3558) (4.6181, 1.326) knots 0 0 0 1 2 2 2
  line L35 (4.6181, 1.326) -> (4.6181, 1.1541)
  line L36 (4.6181, 1.1541) -> (4.6099, 1.1541)
  spline S28 degree 2 poles (4.6099, 1.1541) (4.5481, 1.2035) (4.3979, 1.2601) (4.3207, 1.2601) knots 0 0 0 1 2 2 2
  spline S29 degree 2 poles (4.3207, 1.2601) (4.2415, 1.2601) (4.1324, 1.1932) (4.1324, 1.1263) knots 0 0 0 1 2 2 2
  spline S30 degree 2 poles (4.1324, 1.1263) (4.1324, 1.0656) (4.1972, 1.007) (4.2692, 0.9884) knots 0 0 0 1 2 2 2
  spline S31 degree 2 poles (4.2692, 0.9884) (4.3042, 0.9792) (4.3927, 0.9606) (4.4411, 0.9493) knots 0 0 0 1 2 2 2
  spline S32 degree 2 poles (4.4411, 0.9493) (4.5461, 0.9226) (4.6531, 0.8001) (4.6531, 0.6941) knots 0 0 0 1 2 2 2
  spline S33 degree 2 poles (4.6531, 0.6941) (4.6531, 0.6323) (4.6048, 0.5232) (4.5574, 0.4831) knots 0 0 0 1 2 2 2
  spline S34 degree 2 poles (4.5574, 0.4831) (4.507, 0.4409) (4.3783, 0.3967) (4.2806, 0.3967) knots 0 0 0 1 2 2 2
  spline S35 degree 2 poles (5.0596, 0.3967) (4.9639, 0.3967) (4.7982, 0.4481) (4.7437, 0.4769) knots 0 0 0 1 2 2 2
  line L37 (4.7437, 0.4769) -> (4.7437, 0.657)
  line L38 (4.7437, 0.657) -> (4.7519, 0.657)
  spline S36 degree 2 poles (4.7519, 0.657) (4.7725, 0.6406) (4.8281, 0.6015) (4.8744, 0.5798) knots 0 0 0 1 2 2 2
  spline S37 degree 2 poles (4.8744, 0.5798) (4.9145, 0.5603) (5.0133, 0.5315) (5.0658, 0.5315) knots 0 0 0 1 2 2 2
  spline S38 degree 2 poles (5.0658, 0.5315) (5.1039, 0.5315) (5.1914, 0.549) (5.212, 0.5634) knots 0 0 0 1 2 2 2
  spline S39 degree 2 poles (5.212, 0.5634) (5.2418, 0.5829) (5.2686, 0.6272) (5.2686, 0.6725) knots 0 0 0 1 2 2 2
  spline S40 degree 2 poles (5.2686, 0.6725) (5.2686, 0.7291) (5.2068, 0.7877) (5.1276, 0.8073) knots 0 0 0 1 2 2 2
  spline S41 degree 2 poles (5.1276, 0.8073) (5.0967, 0.8145) (4.9979, 0.8351) (4.9557, 0.8464) knots 0 0 0 1 2 2 2
  spline S42 degree 2 poles (4.9557, 0.8464) (4.8466, 0.8783) (4.7478, 1.01) (4.7478, 1.1037) knots 0 0 0 1 2 2 2
  spline S43 degree 2 poles (4.7478, 1.1037) (4.7478, 1.2334) (4.9423, 1.395) (5.1029, 1.395) knots 0 0 0 1 2 2 2
  spline S44 degree 2 poles (5.1029, 1.395) (5.1821, 1.395) (5.3427, 1.3558) (5.3972, 1.326) knots 0 0 0 1 2 2 2
  line L39 (5.3972, 1.326) -> (5.3972, 1.1541)
  line L40 (5.3972, 1.1541) -> (5.389, 1.1541)
  spline S45 degree 2 poles (5.389, 1.1541) (5.3272, 1.2035) (5.177, 1.2601) (5.0998, 1.2601) knots 0 0 0 1 2 2 2
  spline S46 degree 2 poles (5.0998, 1.2601) (5.0205, 1.2601) (4.9114, 1.1932) (4.9114, 1.1263) knots 0 0 0 1 2 2 2
  spline S47 degree 2 poles (4.9114, 1.1263) (4.9114, 1.0656) (4.9763, 1.007) (5.0483, 0.9884) knots 0 0 0 1 2 2 2
  spline S48 degree 2 poles (5.0483, 0.9884) (5.0833, 0.9792) (5.1718, 0.9606) (5.2202, 0.9493) knots 0 0 0 1 2 2 2
  spline S49 degree 2 poles (5.2202, 0.9493) (5.3252, 0.9226) (5.4322, 0.8001) (5.4322, 0.6941) knots 0 0 0 1 2 2 2
  spline S50 degree 2 poles (5.4322, 0.6941) (5.4322, 0.6323) (5.3838, 0.5232) (5.3365, 0.4831) knots 0 0 0 1 2 2 2
  spline S51 degree 2 poles (5.3365, 0.4831) (5.2861, 0.4409) (5.1574, 0.3967) (5.0596, 0.3967) knots 0 0 0 1 2 2 2
  line L41 (5.7451, 0.4193) -> (5.5845, 0.4193)
  line L42 (5.5845, 0.4193) -> (5.5845, 1.3723)
  line L43 (5.5845, 1.3723) -> (5.7451, 1.3723)
  line L44 (5.7451, 1.3723) -> (5.7451, 0.4193)
  line L45 (5.7564, 1.5308) -> (5.5742, 1.5308)
  line L46 (5.5742, 1.5308) -> (5.5742, 1.6975)
  line L47 (5.5742, 1.6975) -> (5.7564, 1.6975)
  line L48 (5.7564, 1.6975) -> (5.7564, 1.5308)
  spline S52 degree 2 poles (6.764, 0.8958) (6.764, 0.655) (6.5324, 0.3925) (6.3389, 0.3925) knots 0 0 0 1 2 2 2
  spline S53 degree 2 poles (6.3389, 0.3925) (6.1403, 0.3925) (5.9128, 0.6632) (5.9128, 0.8958) knots 0 0 0 1 2 2 2
  spline S54 degree 2 poles (5.9128, 0.8958) (5.9128, 1.1346) (6.1475, 1.3991) (6.3389, 1.3991) knots 0 0 0 1 2 2 2
  spline S55 degree 2 poles (6.3389, 1.3991) (6.5324, 1.3991) (6.764, 1.1356) (6.764, 0.8958) knots 0 0 0 1 2 2 2
  spline S56 degree 2 poles (6.5983, 0.8958) (6.5983, 1.0811) (6.4634, 1.2612) (6.3389, 1.2612) knots 0 0 0 1 2 2 2
  spline S57 degree 2 poles (6.3389, 1.2612) (6.2144, 1.2612) (6.0785, 1.0811) (6.0785, 0.8958) knots 0 0 0 1 2 2 2
  spline S58 degree 2 poles (6.0785, 0.8958) (6.0785, 0.7157) (6.2144, 0.5304) (6.3389, 0.5304) knots 0 0 0 1 2 2 2
  spline S59 degree 2 poles (6.3389, 0.5304) (6.4624, 0.5304) (6.5983, 0.7126) (6.5983, 0.8958) knots 0 0 0 1 2 2 2
  line L49 (7.6768, 0.4193) -> (7.5163, 0.4193)
  line L50 (7.5163, 0.4193) -> (7.5163, 0.9627)
  spline S60 degree 2 poles (7.5163, 0.9627) (7.5163, 1.0286) (7.5039, 1.1418) (7.4854, 1.1757) knots 0 0 0 1 2 2 2
  spline S61 degree 2 poles (7.4854, 1.1757) (7.4659, 1.2118) (7.3959, 1.2468) (7.3362, 1.2468) knots 0 0 0 1 2 2 2
  spline S62 degree 2 poles (7.3362, 1.2468) (7.2765, 1.2468) (7.1499, 1.1829) (7.0892, 1.1315) knots 0 0 0 1 2 2 2
  line L51 (7.0892, 1.1315) -> (7.0892, 0.4193)
  line L52 (7.0892, 0.4193) -> (6.9286, 0.4193)
  line L53 (6.9286, 0.4193) -> (6.9286, 1.3723)
  line L54 (6.9286, 1.3723) -> (7.0892, 1.3723)
  line L55 (7.0892, 1.3723) -> (7.0892, 1.2663)
  spline S63 degree 2 poles (7.0892, 1.2663) (7.1612, 1.3311) (7.3002, 1.3991) (7.3784, 1.3991) knots 0 0 0 1 2 2 2
  spline S64 degree 2 poles (7.3784, 1.3991) (7.5183, 1.3991) (7.6768, 1.2138) (7.6768, 1.0378) knots 0 0 0 1 2 2 2
  line L56 (7.6768, 1.0378) -> (7.6768, 0.4193)
  spline S65 degree 2 poles (8.8141, 0.3967) (8.6762, 0.3967) (8.4827, 0.4543) (8.3973, 0.4955) knots 0 0 0 1 2 2 2
  line L57 (8.3973, 0.4955) -> (8.3973, 0.7075)
  line L58 (8.3973, 0.7075) -> (8.4096, 0.7075)
  spline S66 degree 2 poles (8.4096, 0.7075) (8.493, 0.6292) (8.7039, 0.5428) (8.8017, 0.5428) knots 0 0 0 1 2 2 2
  spline S67 degree 2 poles (8.8017, 0.5428) (8.9417, 0.5428) (9.0847, 0.6591) (9.0847, 0.7548) knots 0 0 0 1 2 2 2
  spline S68 degree 2 poles (9.0847, 0.7548) (9.0847, 0.831) (9.0096, 0.9257) (8.9283, 0.9493) knots 0 0 0 1 2 2 2
  spline S69 degree 2 poles (8.9283, 0.9493) (8.8696, 0.9658) (8.7719, 0.9884) (8.6988, 1.007) knots 0 0 0 1 2 2 2
  spline S70 degree 2 poles (8.6988, 1.007) (8.6329, 1.0245) (8.529, 1.0769) (8.4889, 1.1191) knots 0 0 0 1 2 2 2
  spline S71 degree 2 poles (8.4889, 1.1191) (8.4497, 1.1613) (8.4065, 1.2745) (8.4065, 1.3486) knots 0 0 0 1 2 2 2
  spline S72 degree 2 poles (8.4065, 1.3486) (8.4065, 1.503) (8.6473, 1.7119) (8.8336, 1.7119) knots 0 0 0 1 2 2 2
  spline S73 degree 2 poles (8.8336, 1.7119) (8.9407, 1.7119) (9.13, 1.6697) (9.2113, 1.6296) knots 0 0 0 1 2 2 2
  line L59 (9.2113, 1.6296) -> (9.2113, 1.4279)
  line L60 (9.2113, 1.4279) -> (9.199, 1.4279)
  spline S74 degree 2 poles (9.199, 1.4279) (9.1383, 1.4835) (8.9489, 1.5658) (8.8449, 1.5658) knots 0 0 0 1 2 2 2
  spline S75 degree 2 poles (8.8449, 1.5658) (8.7276, 1.5658) (8.5825, 1.4557) (8.5825, 1.3661) knots 0 0 0 1 2 2 2
  spline S76 degree 2 poles (8.5825, 1.3661) (8.5825, 1.2859) (8.6679, 1.1901) (8.7482, 1.1685) knots 0 0 0 1 2 2 2
  spline S77 degree 2 poles (8.7482, 1.1685) (8.8017, 1.1541) (8.9571, 1.1171) (9.0086, 1.1016) knots 0 0 0 1 2 2 2
  spline S78 degree 2 poles (9.0086, 1.1016) (9.1393, 1.0615) (9.2607, 0.8999) (9.2607, 0.7816) knots 0 0 0 1 2 2 2
  spline S79 degree 2 poles (9.2607, 0.7816) (9.2607, 0.7064) (9.2, 0.5624) (9.1455, 0.5119) knots 0 0 0 1 2 2 2
  spline S80 degree 2 poles (9.1455, 0.5119) (9.0847, 0.4563) (8.9304, 0.3967) (8.8141, 0.3967) knots 0 0 0 1 2 2 2
  spline S81 degree 2 poles (9.9513, 0.5202) (9.9318, 0.5057) (9.8659, 0.4543) (9.835, 0.4389) knots 0 0 0 1 2 2 2
  spline S82 degree 2 poles (9.835, 0.4389) (9.7928, 0.4162) (9.7136, 0.3925) (9.6415, 0.3925) knots 0 0 0 1 2 2 2
  spline S83 degree 2 poles (9.6415, 0.3925) (9.5829, 0.3925) (9.4769, 0.4368) (9.4367, 0.4769) knots 0 0 0 1 2 2 2
  spline S84 degree 2 poles (9.4367, 0.4769) (9.3986, 0.516) (9.3523, 0.6313) (9.3523, 0.6951) knots 0 0 0 1 2 2 2
  spline S85 degree 2 poles (9.3523, 0.6951) (9.3523, 0.7939) (9.4357, 0.9339) (9.5263, 0.974) knots 0 0 0 1 2 2 2
  spline S86 degree 2 poles (9.5263, 0.974) (9.6065, 1.0111) (9.8247, 1.0389) (9.9513, 1.0461) knots 0 0 0 1 2 2 2
  line L61 (9.9513, 1.0461) -> (9.9513, 1.0769)
  spline S87 degree 2 poles (9.9513, 1.0769) (9.9513, 1.1325) (9.9173, 1.2015) (9.8865, 1.221) knots 0 0 0 1 2 2 2
  spline S88 degree 2 poles (9.8865, 1.221) (9.8556, 1.2406) (9.7671, 1.2529) (9.7197, 1.2529) knots 0 0 0 1 2 2 2
  spline S89 degree 2 poles (9.7197, 1.2529) (9.6642, 1.2529) (9.5139, 1.22) (9.4388, 1.1881) knots 0 0 0 1 2 2 2
  line L62 (9.4388, 1.1881) -> (9.4295, 1.1881)
  line L63 (9.4295, 1.1881) -> (9.4295, 1.3517)
  spline S90 degree 2 poles (9.4295, 1.3517) (9.4738, 1.3641) (9.6395, 1.395) (9.7208, 1.395) knots 0 0 0 1 2 2 2
  spline S91 degree 2 poles (9.7208, 1.395) (9.8196, 1.395) (9.9544, 1.3641) (10.0079, 1.3239) knots 0 0 0 1 2 2 2
  spline S92 degree 2 poles (10.0079, 1.3239) (10.0604, 1.2848) (10.1119, 1.1603) (10.1119, 1.0708) knots 0 0 0 1 2 2 2
  line L64 (10.1119, 1.0708) -> (10.1119, 0.4193)
  line L65 (10.1119, 0.4193) -> (9.9513, 0.4193)
  line L66 (9.9513, 0.4193) -> (9.9513, 0.5202)
  line L67 (9.9513, 0.6539) -> (9.9513, 0.9184)
  spline S93 degree 2 poles (9.9513, 0.9184) (9.8937, 0.9133) (9.7197, 0.8958) (9.6652, 0.8793) knots 0 0 0 1 2 2 2
  spline S94 degree 2 poles (9.6652, 0.8793) (9.6014, 0.8598) (9.518, 0.7785) (9.518, 0.7064) knots 0 0 0 1 2 2 2
  spline S95 degree 2 poles (9.518, 0.7064) (9.518, 0.6241) (9.6107, 0.5407) (9.6992, 0.5407) knots 0 0 0 1 2 2 2
  spline S96 degree 2 poles (9.6992, 0.5407) (9.7743, 0.5407) (9.8978, 0.6056) (9.9513, 0.6539) knots 0 0 0 1 2 2 2
  line L68 (11.0855, 0.4193) -> (10.9249, 0.4193)
  line L69 (10.9249, 0.4193) -> (10.9249, 0.9627)
  spline S97 degree 2 poles (10.9249, 0.9627) (10.9249, 1.0286) (10.9126, 1.1418) (10.894, 1.1757) knots 0 0 0 1 2 2 2
  spline S98 degree 2 poles (10.894, 1.1757) (10.8745, 1.2118) (10.8045, 1.2468) (10.7448, 1.2468) knots 0 0 0 1 2 2 2
  spline S99 degree 2 poles (10.7448, 1.2468) (10.6851, 1.2468) (10.5585, 1.1829) (10.4978, 1.1315) knots 0 0 0 1 2 2 2
  line L70 (10.4978, 1.1315) -> (10.4978, 0.4193)
  line L71 (10.4978, 0.4193) -> (10.3372, 0.4193)
  line L72 (10.3372, 0.4193) -> (10.3372, 1.3723)
  line L73 (10.3372, 1.3723) -> (10.4978, 1.3723)
  line L74 (10.4978, 1.3723) -> (10.4978, 1.2663)
  spline S100 degree 2 poles (10.4978, 1.2663) (10.5698, 1.3311) (10.7088, 1.3991) (10.787, 1.3991) knots 0 0 0 1 2 2 2
  spline S101 degree 2 poles (10.787, 1.3991) (10.927, 1.3991) (11.0855, 1.2138) (11.0855, 1.0378) knots 0 0 0 1 2 2 2
  line L75 (11.0855, 1.0378) -> (11.0855, 0.4193)
  spline S102 degree 2 poles (12.3472, 0.7497) (12.3472, 0.5829) (12.1434, 0.4018) (11.9716, 0.4018) knots 0 0 0 1 2 2 2
  spline S103 degree 2 poles (11.9716, 0.4018) (11.9304, 0.4018) (11.7935, 0.4162) (11.7472, 0.4265) knots 0 0 0 1 2 2 2
  line L76 (11.7472, 0.4265) -> (11.7472, 0.5891)
  line L77 (11.7472, 0.5891) -> (11.7565, 0.5891)
  spline S104 degree 2 poles (11.7565, 0.5891) (11.7915, 0.5768) (11.8954, 0.5479) (11.9489, 0.5479) knots 0 0 0 1 2 2 2
  spline S105 degree 2 poles (11.9489, 0.5479) (12.0272, 0.5479) (12.1208, 0.584) (12.1424, 0.6169) knots 0 0 0 1 2 2 2
  spline S106 degree 2 poles (12.1424, 0.6169) (12.1661, 0.6509) (12.1784, 0.7497) (12.1784, 0.8145) knots 0 0 0 1 2 2 2
  line L78 (12.1784, 0.8145) -> (12.1784, 1.5545)
  line L79 (12.1784, 1.5545) -> (11.9098, 1.5545)
  line L80 (11.9098, 1.5545) -> (11.9098, 1.6893)
  line L81 (11.9098, 1.6893) -> (12.3472, 1.6893)
  line L82 (12.3472, 1.6893) -> (12.3472, 0.7497)
  spline S107 degree 2 poles (13.3671, 0.8958) (13.3671, 0.655) (13.1356, 0.3925) (12.9421, 0.3925) knots 0 0 0 1 2 2 2
  spline S108 degree 2 poles (12.9421, 0.3925) (12.7435, 0.3925) (12.516, 0.6632) (12.516, 0.8958) knots 0 0 0 1 2 2 2
  spline S109 degree 2 poles (12.516, 0.8958) (12.516, 1.1346) (12.7507, 1.3991) (12.9421, 1.3991) knots 0 0 0 1 2 2 2
  spline S110 degree 2 poles (12.9421, 1.3991) (13.1356, 1.3991) (13.3671, 1.1356) (13.3671, 0.8958) knots 0 0 0 1 2 2 2
  spline S111 degree 2 poles (13.2014, 0.8958) (13.2014, 1.0811) (13.0666, 1.2612) (12.9421, 1.2612) knots 0 0 0 1 2 2 2
  spline S112 degree 2 poles (12.9421, 1.2612) (12.8176, 1.2612) (12.6817, 1.0811) (12.6817, 0.8958) knots 0 0 0 1 2 2 2
  spline S113 degree 2 poles (12.6817, 0.8958) (12.6817, 0.7157) (12.8176, 0.5304) (12.9421, 0.5304) knots 0 0 0 1 2 2 2
  spline S114 degree 2 poles (12.9421, 0.5304) (13.0656, 0.5304) (13.2014, 0.7126) (13.2014, 0.8958) knots 0 0 0 1 2 2 2
  spline S115 degree 2 poles (13.7891, 0.3967) (13.6934, 0.3967) (13.5277, 0.4481) (13.4731, 0.4769) knots 0 0 0 1 2 2 2
  line L83 (13.4731, 0.4769) -> (13.4731, 0.657)
  line L84 (13.4731, 0.657) -> (13.4814, 0.657)
  spline S116 degree 2 poles (13.4814, 0.657) (13.502, 0.6406) (13.5575, 0.6015) (13.6038, 0.5798) knots 0 0 0 1 2 2 2
  spline S117 degree 2 poles (13.6038, 0.5798) (13.644, 0.5603) (13.7428, 0.5315) (13.7953, 0.5315) knots 0 0 0 1 2 2 2
  spline S118 degree 2 poles (13.7953, 0.5315) (13.8334, 0.5315) (13.9208, 0.549) (13.9414, 0.5634) knots 0 0 0 1 2 2 2
  spline S119 degree 2 poles (13.9414, 0.5634) (13.9713, 0.5829) (13.998, 0.6272) (13.998, 0.6725) knots 0 0 0 1 2 2 2
  spline S120 degree 2 poles (13.998, 0.6725) (13.998, 0.7291) (13.9363, 0.7877) (13.857, 0.8073) knots 0 0 0 1 2 2 2
  spline S121 degree 2 poles (13.857, 0.8073) (13.8261, 0.8145) (13.7273, 0.8351) (13.6851, 0.8464) knots 0 0 0 1 2 2 2
  spline S122 degree 2 poles (13.6851, 0.8464) (13.5761, 0.8783) (13.4773, 1.01) (13.4773, 1.1037) knots 0 0 0 1 2 2 2
  spline S123 degree 2 poles (13.4773, 1.1037) (13.4773, 1.2334) (13.6718, 1.395) (13.8323, 1.395) knots 0 0 0 1 2 2 2
  spline S124 degree 2 poles (13.8323, 1.395) (13.9116, 1.395) (14.0721, 1.3558) (14.1267, 1.326) knots 0 0 0 1 2 2 2
  line L85 (14.1267, 1.326) -> (14.1267, 1.1541)
  line L86 (14.1267, 1.1541) -> (14.1184, 1.1541)
  spline S125 degree 2 poles (14.1184, 1.1541) (14.0567, 1.2035) (13.9064, 1.2601) (13.8292, 1.2601) knots 0 0 0 1 2 2 2
  spline S126 degree 2 poles (13.8292, 1.2601) (13.75, 1.2601) (13.6409, 1.1932) (13.6409, 1.1263) knots 0 0 0 1 2 2 2
  spline S127 degree 2 poles (13.6409, 1.1263) (13.6409, 1.0656) (13.7057, 1.007) (13.7778, 0.9884) knots 0 0 0 1 2 2 2
  spline S128 degree 2 poles (13.7778, 0.9884) (13.8128, 0.9792) (13.9013, 0.9606) (13.9496, 0.9493) knots 0 0 0 1 2 2 2
  spline S129 degree 2 poles (13.9496, 0.9493) (14.0546, 0.9226) (14.1617, 0.8001) (14.1617, 0.6941) knots 0 0 0 1 2 2 2
  spline S130 degree 2 poles (14.1617, 0.6941) (14.1617, 0.6323) (14.1133, 0.5232) (14.0659, 0.4831) knots 0 0 0 1 2 2 2
  spline S131 degree 2 poles (14.0659, 0.4831) (14.0155, 0.4409) (13.8869, 0.3967) (13.7891, 0.3967) knots 0 0 0 1 2 2 2
  spline S132 degree 2 poles (14.7246, 0.3977) (14.4961, 0.3977) (14.245, 0.6539) (14.245, 0.8907) knots 0 0 0 1 2 2 2
  spline S133 degree 2 poles (14.245, 0.8907) (14.245, 1.1233) (14.4889, 1.3991) (14.6855, 1.3991) knots 0 0 0 1 2 2 2
  spline S134 degree 2 poles (14.6855, 1.3991) (14.774, 1.3991) (14.9109, 1.3476) (14.9613, 1.2931) knots 0 0 0 1 2 2 2
  spline S135 degree 2 poles (14.9613, 1.2931) (15.0128, 1.2385) (15.0673, 1.0811) (15.0673, 0.9668) knots 0 0 0 1 2 2 2
  line L87 (15.0673, 0.9668) -> (15.0673, 0.8793)
  line L88 (15.0673, 0.8793) -> (14.4076, 0.8793)
  spline S136 degree 2 poles (14.4076, 0.8793) (14.4076, 0.7136) (14.5744, 0.5377) (14.7226, 0.5377) knots 0 0 0 1 2 2 2
  spline S137 degree 2 poles (14.7226, 0.5377) (14.775, 0.5377) (14.8769, 0.5613) (14.9181, 0.5798) knots 0 0 0 1 2 2 2
  spline S138 degree 2 poles (14.9181, 0.5798) (14.9613, 0.6004) (15.021, 0.6365) (15.0406, 0.6529) knots 0 0 0 1 2 2 2